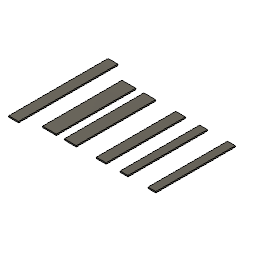
Skeleton (Autodesk Fusion 360 design; units mm, degrees)
part number: 2026-01-13-13-52-06-648
Autodesk Fusion 360 part; units mm, degrees
sketch "Sketch1" plane through (0, 0, 0) normal (0, 0, 1) x (1, 0, 0)
sketch "Sketch2" plane through (0, 0, 0) normal (0, 0, 1) x (1, 0, 0)
  line L0 (-35, 200) -> (0, 200)
  line L1 (0, 200) -> (0, 0)
  line L2 (0, 0) -> (-35, 0)
  line L3 (-35, 0) -> (-35, 200)
  line L4 (20, 200) -> (50, 200)
  line L5 (50, 200) -> (50, 0)
  line L6 (50, 0) -> (20, 0)
  line L7 (20, 0) -> (20, 200)
  line L8 (100, 200) -> (125, 200)
  line L9 (125, 200) -> (125, 0)
  line L10 (125, 0) -> (100, 0)
  line L11 (100, 0) -> (100, 200)
  line L12 (160, 200) -> (180, 200)
  line L13 (180, 200) -> (180, 0)
  line L14 (180, 0) -> (160, 0)
  line L15 (160, 0) -> (160, 200)
  line L16 (230, 200) -> (250, 200)
  line L17 (250, 200) -> (250, 0)
  line L18 (250, 0) -> (230, 0)
  line L19 (230, 0) -> (230, 200)
  dimension "d1" = 200
  dimension "d2" = 35
  dimension "d3" = 30
  dimension "d4" = 200
  dimension "d5" = 25
  dimension "d6" = 20
  dimension "d7" = 20
  dimension "d8" = 200
  dimension "d9" = 200
  dimension "d10" = 200
  constraint horizontal L0
  constraint vertical L1
  constraint horizontal L2
  constraint vertical L3
  constraint coincident L1.end L2.start
  constraint horizontal L4
  constraint vertical L5
  constraint horizontal L6
  constraint vertical L7
  constraint horizontal L8
  constraint vertical L9
  constraint horizontal L10
  constraint vertical L11
  constraint horizontal L12
  constraint vertical L13
  constraint horizontal L14
  constraint vertical L15
  constraint horizontal L16
  constraint vertical L17
  constraint horizontal L18
  constraint vertical L19
  measures "d1" distance of L0.start L2.end
  measures "d2" distance of L0.start L0.end
  measures "d3" distance of L4.start L4.end
  measures "d4" distance of L4.end L5.end
  measures "d5" distance of L8.start L8.end
  measures "d6" distance of L12.start L12.end
  measures "d7" distance of L16.start L16.end
  measures "d8" distance of L8.end L9.end
  measures "d9" distance of L12.end L13.end
  measures "d10" distance of L16.end L17.end
extrude "Extrude1" add sketch "Sketch2" along normal blind 3 makes body 1 at (108.3333, 66.6667, 0) makes body 2 at (30, 133.3333, 0) makes body 3 at (166.6667, 133.3333, 0) makes body 4 at (-23.3333, 133.3333, 0) makes body 5 at (236.6667, 66.6667, 0)
sketch "Sketch3" plane through (0, 0, 0) normal (0, 0, 1) x (1, 0, 0)
  line L0 (-100, 230) -> (-75, 230)
  line L1 (-75, 230) -> (-75, -20)
  line L2 (-75, -20) -> (-100, -20)
  line L3 (-100, -20) -> (-100, 230)
  dimension "d13" = 25
  dimension "d14" = 250
  constraint horizontal L0
  constraint vertical L1
  constraint horizontal L2
  constraint vertical L3
  measures "d13" distance of L0.start L0.end
  measures "d14" distance of L0.end L1.end
extrude "Extrude2" add sketch "Sketch3" along normal blind 3 separate body makes body 6
